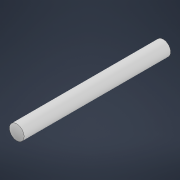
# Autodesk Inventor part: Poker hinge 3
Saved by Autodesk Inventor 2022 (Build 260153000, 153)
## iProperties
Created: 2021-05-25
Part Number: Poker hinge 3
Material: Generic
Document SubType Name: Modeling
Designer: Albert L Tomberg
Density: 1 g/cm^3
Appearance: Default
Author: Albert L Tomberg
Autodesk Inventor part; units mm, degrees
ref_plane "YZ Plane" through (0, 0, 0) normal (1, 0, 0) x (0, 1, 0)
ref_plane "XZ Plane" through (0, 0, 0) normal (0, 1, 0) x (-1, 0, 0)
ref_plane "XY Plane" through (0, 0, 0) normal (0, 0, 1) x (1, 0, 0)
sketch "Sketch1" plane through (0, 0, 0) normal (0, 0, 1) x (1, 0, 0)
  circle A0 centre (0, 0) radius 2
  dimension "d0" = 4
  constraints: 1 centre point, 1 coincident
  measures "d0" diameter of A0
extrude "Extrusion1" add sketch "Sketch1" against normal blind 40
sketch "Sketch3" plane through (0, 0, 0) normal (1, 0, 0) x (0, 1, 0)
  line L0 (0, 0) -> (0, 0.5)
  line L1 (2, 0) -> (-2, 0) projected
  arc A0 (2, 0) -> (0, 0.5) centre (0, -3.75) ccw
  line L2 (2, 0) -> (0, 0)
  dimension "d5" = 0.5
  dimension "d7" = 4.25
  constraints: 4 end point, 2 point on circle, 1 centre point, 1 collinear, 1 vertical
  measures "d5" distance of L0.start L0.end
  measures "d7" radius of A0
revolve "Revolution1" add sketch "Sketch3" angle 360 about axis through (0, 0, 0) along (0, 0, 1)
sketch "Sketch4" plane through (0, 0, 0) normal (1, 0, 0) x (0, 1, 0)
  line L0 (-2, -40) -> (2, -40) projected
  line L1 (0, -40) -> (0, -40.5)
  arc A0 (0, -40.5) -> (2, -40) centre (0, -36.25) ccw
  line L2 (2, -40) -> (0, -40)
  point P0 (0, 0)
  dimension "d9" = 0.5
  dimension "d11" = 4.25
  constraints: 4 end point, 2 point on circle, 1 centre point, 1 midpoint, 1 perpendicular, 1 vertical
  measures "d9" distance of L1.start L1.end
  measures "d11" radius of A0
revolve "Revolution2" add sketch "Sketch4" angle 360 about axis through (0, 0, -40) along (0, 0, -1)
body "Solid1"
